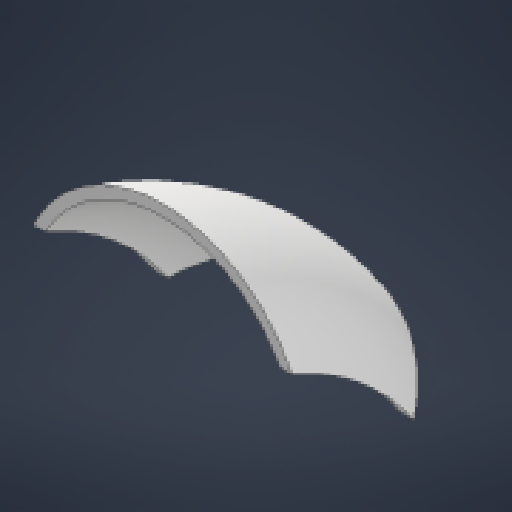
# Autodesk Inventor part: изменение траектории 25-26
Saved by Autodesk Inventor 2025 (Build 290162000, 162)
## iProperties
Created: 2025-11-02
Part Number: изменение траектории 25-26
Material: Типовые
Document SubType Name: Modeling
Designer: Phantom
Density: 1 g/cm^3
Appearance: По умолчанию
Author: Phantom
Autodesk Inventor part; units mm, degrees
ref_plane "YZ Plane" through (0, 0, 0) normal (1, 0, 0) x (0, 1, 0)
ref_plane "XZ Plane" through (0, 0, 0) normal (0, 1, 0) x (-1, 0, 0)
ref_plane "XY Plane" through (0, 0, 0) normal (0, 0, 1) x (1, 0, 0)
sketch "Эскиз1" plane through (0, 0, 0) normal (0, 0, 1) x (1, 0, 0)
  circle A0 centre (0, 0) radius 63.5
  circle A1 centre (0, 0) radius 68.5
  line L0 (-68.5, 0) -> (68.5, 0)
  point P0 (-63.5, 0)
  point P1 (63.5, 0)
  dimension "d0" = 127
  dimension "d1" = 137
  constraints: 2 centre point, 2 coincident, 2 end point, 2 point on circle, 1 horizontal
  measures "d0" diameter of A0
  measures "d1" diameter of A1
sketch "Эскиз2" plane through (0, 0, 0) normal (1, 0, 0) x (0, 1, 0)
  line L0 (0, 0) -> (-98, 0)
  arc A0 (-98, -180) -> (51.4499, -100.3231) centre (-98, 0) ccw
  line L1 (63.5, 0) -> (-63.5, 0) projected
  dimension "d6" = 360
  dimension "d7" = 98
  constraints: 2 end point, 2 point on circle, 1 centre point, 1 coincident, 1 horizontal, 1 midpoint
  measures "d6" diameter of A0
  measures "d7" distance of A0.centre point (0, 0)
sweep "Сдвиг2" add profiles "Эскиз1" path "Эскиз2" picked at (5.5611, 64.7671) path curves A0 contours A0 L0 A1
sketch "Эскиз3" plane through (0, 0, 0) normal (1, 0, 0) x (0, 1, 0)
  line L0 (21.671, -50.7823) -> (67.1006, -50.7823) projected
  line L1 (21.671, -50.7823) -> (-49.0926, -50.7823)
  line L2 (-49.0926, -50.7823) -> (124.8994, -50.7823)
  line L3 (124.8994, -50.7823) -> (124.8994, 54.6872)
  line L4 (124.8994, 54.6872) -> (-32.5885, 54.6872)
  line L5 (-32.5885, 54.6872) -> (-49.0926, -50.7823)
  point P0 (0, 0)
  constraints: 10 end point, 2 perpendicular, 1 horizontal, 1 point on line
extrude "Выдавливание1" cut sketch "Эскиз3" along normal through all both and the other way through all
sketch "Эскиз4" plane through (0, 0, 0) normal (1, 0, 0) x (0, 1, 0)
  arc A0 (21.671, -50.7823) -> (-109.914, 129.4529) centre (-98, 0) ccw projected
  circle A1 centre (-98, 0) radius 130
  arc A2 (-43.3796, -81.3672) -> (0, 0) centre (-98, 0) ccw projected
  point P0 (-14.1838, -50.7823)
  point P1 (-109.914, 129.4529)
  point P2 (21.671, -50.7823)
  constraints: 1 centre point, 1 coincident, 1 concentric
ref_plane "РабПлоскость1" through (-60.5707, -122.8992, 62.7178) normal (1, 0, 0) x (0, -1, 0)
sketch "Эскиз5" plane through (-60.5707, -122.8992, 62.7178) normal (1, 0, 0) x (0, -1, 0)
  point P0 (-122.8992, 62.7178)
